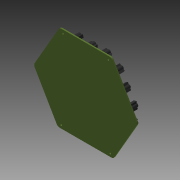
# Autodesk Inventor part: PCB
Saved by Autodesk Inventor 2015 (Build 190159000, 159)
## iProperties
Created: 2016-10-01
Part Number: PCB
Material: Generic
Document SubType Name: Modeling
Designer: James Yelland
Density: 1 g/cm^3
Appearance: Default
Author: James Yelland
Autodesk Inventor part; units mm, degrees
ref_plane "YZ Plane" through (0, 0, 0) normal (1, 0, 0) x (0, 1, 0)
ref_plane "XZ Plane" through (0, 0, 0) normal (0, 1, 0) x (-1, 0, 0)
ref_plane "XY Plane" through (0, 0, 0) normal (0, 0, 1) x (1, 0, 0)
sketch "Sketch1" plane through (0, 0, 0) normal (0, 1, 0) x (-1, 0, 0)
  line L0 (-78.5566, 2.5) -> (-41.4434, 66.782)
  line L1 (-37.1132, 69.282) -> (37.1132, 69.282)
  line L2 (41.4434, 66.782) -> (78.5566, 2.5)
  line L3 (0, -64.282) -> (-40, -64.282)
  line L4 (0, -64.282) -> (40, -64.282)
  line L5 (78.5566, -2.5) -> (44.3301, -61.782)
  line L6 (-44.3301, -61.782) -> (-78.5566, -2.5)
  arc A0 (78.5566, -2.5) -> (78.5566, 2.5) centre (74.2265, 0) ccw
  arc A1 (40, -64.282) -> (44.3301, -61.782) centre (40, -59.282) ccw
  arc A2 (-44.3301, -61.782) -> (-40, -64.282) centre (-40, -59.282) ccw
  arc A3 (-78.5566, 2.5) -> (-78.5566, -2.5) centre (-74.2265, 0) ccw
  arc A4 (-37.1132, 69.282) -> (-41.4434, 66.782) centre (-37.1132, 64.282) ccw
  arc A5 (41.4434, 66.782) -> (37.1132, 69.282) centre (37.1132, 64.282) ccw
  circle A6 centre (37.937, -59.3323) radius 1.6
  circle A7 centre (-37.937, -59.3323) radius 1.6
  circle A8 centre (-35.0503, 64.3323) radius 1.6
  circle A9 centre (35.0503, 64.3323) radius 1.6
  point P0 (80, 0)
  point P1 (-80, 0)
  point P2 (-42.8868, -64.282)
  point P3 (42.8868, -64.282)
  dimension "d21" = 5
  dimension "d35" = 3.2
  dimension "d38" = 3.2
  dimension "d45" = 3.2
  dimension "d46" = 3.2
  constraints: 14 end point, 12 point on circle, 12 tangent, 10 centre point, 9 point on line, 5 equal radius
  measures "d21" radius of A0
  measures "d35" diameter of A6
  measures "d38" diameter of A7
  measures "d45" diameter of A8
  measures "d46" diameter of A9
extrude "Extrusion1" add sketch "Sketch1" along normal blind 2
sketch "Sketch4" plane through (0, 2, 0) normal (0, 1, 0) x (1, 0, 0)
  line L0 (5, 57.282) -> (5, 53.282)
  arc A0 (2.5807, 57.282) -> (-2.5807, 57.282) centre (0, 56.332) ccw
  line L1 (-5, 57.282) -> (-2.5807, 57.282)
  line L2 (5, 53.282) -> (-5, 53.282)
  line L3 (-5, 53.282) -> (-5, 57.282)
  line L4 (2.5807, 57.282) -> (5, 57.282)
  line L5 (-24.333, 52.2353) -> (-25.7011, 55.9941)
  line L6 (-25.7011, 55.9941) -> (-23.4277, 56.8215)
  arc A1 (-18.5775, 58.5868) -> (-23.4277, 56.8215) centre (-20.6777, 56.8115) ccw
  line L7 (-14.9361, 55.6555) -> (-24.333, 52.2353)
  line L8 (-16.3041, 59.4143) -> (-14.9361, 55.6555)
  line L9 (-18.5775, 58.5868) -> (-16.3041, 59.4143)
  line L10 (-44.1513, 44.8388) -> (-46.7224, 47.903)
  line L11 (-46.7224, 47.903) -> (-44.8691, 49.4581)
  arc A2 (-40.9153, 52.7758) -> (-44.8691, 49.4581) centre (-42.2815, 50.3892) ccw
  line L12 (-36.4908, 51.2667) -> (-44.1513, 44.8388)
  line L13 (-39.062, 54.3309) -> (-36.4908, 51.2667)
  line L14 (-40.9153, 52.7758) -> (-39.062, 54.3309)
  line L15 (-52.9737, 24.8109) -> (-56.4378, 26.8109)
  line L16 (-56.4378, 26.8109) -> (-55.2282, 28.9061)
  arc A3 (-52.6475, 33.376) -> (-55.2282, 28.9061) centre (-53.1151, 30.666) ccw
  line L17 (-47.9737, 33.4711) -> (-52.9737, 24.8109)
  line L18 (-51.4378, 35.4711) -> (-47.9737, 33.4711)
  line L19 (-52.6475, 33.376) -> (-51.4378, 35.4711)
  line L20 (-62.6437, 5.9686) -> (-66.5829, 6.6632)
  line L21 (-66.5829, 6.6632) -> (-66.1628, 9.0458)
  arc A4 (-65.2665, 14.1288) -> (-66.1628, 9.0458) centre (-64.7791, 11.4223) ccw
  line L22 (-60.9072, 15.8167) -> (-62.6437, 5.9686)
  line L23 (-64.8464, 16.5113) -> (-60.9072, 15.8167)
  line L24 (-65.2665, 14.1288) -> (-64.8464, 16.5113)
  line L25 (-60.9072, -15.8167) -> (-64.8464, -16.5113)
  line L26 (-64.8464, -16.5113) -> (-65.2665, -14.1288)
  arc A5 (-66.1628, -9.0458) -> (-65.2665, -14.1288) centre (-64.7791, -11.4223) ccw
  line L27 (-62.6437, -5.9686) -> (-60.9072, -15.8167)
  line L28 (-66.5829, -6.6632) -> (-62.6437, -5.9686)
  line L29 (-66.1628, -9.0458) -> (-66.5829, -6.6632)
  line L30 (-47.9737, -33.4711) -> (-51.4378, -35.4711)
  line L31 (-51.4378, -35.4711) -> (-52.6475, -33.376)
  arc A6 (-55.2282, -28.9061) -> (-52.6475, -33.376) centre (-53.1151, -30.666) ccw
  line L32 (-52.9737, -24.8109) -> (-47.9737, -33.4711)
  line L33 (-56.4378, -26.8109) -> (-52.9737, -24.8109)
  line L34 (-55.2282, -28.9061) -> (-56.4378, -26.8109)
  line L35 (-36.4908, -51.2667) -> (-39.062, -54.3309)
  line L36 (-39.062, -54.3309) -> (-40.9153, -52.7758)
  arc A7 (-44.8691, -49.4581) -> (-40.9153, -52.7758) centre (-42.2815, -50.3892) ccw
  line L37 (-44.1513, -44.8388) -> (-36.4908, -51.2667)
  line L38 (-46.7224, -47.903) -> (-44.1513, -44.8388)
  line L39 (-44.8691, -49.4581) -> (-46.7224, -47.903)
  line L40 (-16.7559, -60.6555) -> (-18.124, -64.4143)
  line L41 (-18.124, -64.4143) -> (-20.3974, -63.5868)
  arc A8 (-25.2475, -61.8215) -> (-20.3974, -63.5868) centre (-22.4975, -61.8115) ccw
  line L42 (-26.1528, -57.2353) -> (-16.7559, -60.6555)
  line L43 (-27.5209, -60.9941) -> (-26.1528, -57.2353)
  line L44 (-25.2475, -61.8215) -> (-27.5209, -60.9941)
  line L45 (5, -58.282) -> (5, -62.282)
  line L46 (5, -62.282) -> (2.5807, -62.282)
  arc A9 (-2.5807, -62.282) -> (2.5807, -62.282) centre (0, -61.332) ccw
  line L47 (-5, -58.282) -> (5, -58.282)
  line L48 (-5, -62.282) -> (-5, -58.282)
  line L49 (-2.5807, -62.282) -> (-5, -62.282)
  line L50 (26.1528, -57.2353) -> (27.5209, -60.9941)
  line L51 (27.5209, -60.9941) -> (25.2475, -61.8215)
  arc A10 (20.3974, -63.5868) -> (25.2475, -61.8215) centre (22.4975, -61.8115) ccw
  line L52 (16.7559, -60.6555) -> (26.1528, -57.2353)
  line L53 (18.124, -64.4143) -> (16.7559, -60.6555)
  line L54 (20.3974, -63.5868) -> (18.124, -64.4143)
  line L55 (44.1513, -44.8388) -> (46.7224, -47.903)
  line L56 (46.7224, -47.903) -> (44.8691, -49.4581)
  arc A11 (40.9153, -52.7758) -> (44.8691, -49.4581) centre (42.2815, -50.3892) ccw
  line L57 (36.4908, -51.2667) -> (44.1513, -44.8388)
  line L58 (39.062, -54.3309) -> (36.4908, -51.2667)
  line L59 (40.9153, -52.7758) -> (39.062, -54.3309)
  line L60 (52.9737, -24.8109) -> (56.4378, -26.8109)
  line L61 (56.4378, -26.8109) -> (55.2282, -28.9061)
  arc A12 (52.6475, -33.376) -> (55.2282, -28.9061) centre (53.1151, -30.666) ccw
  line L62 (47.9737, -33.4711) -> (52.9737, -24.8109)
  line L63 (51.4378, -35.4711) -> (47.9737, -33.4711)
  line L64 (52.6475, -33.376) -> (51.4378, -35.4711)
  line L65 (62.6437, -5.9686) -> (66.5829, -6.6632)
  line L66 (66.5829, -6.6632) -> (66.1628, -9.0458)
  arc A13 (65.2665, -14.1288) -> (66.1628, -9.0458) centre (64.7791, -11.4223) ccw
  line L67 (60.9072, -15.8167) -> (62.6437, -5.9686)
  line L68 (64.8464, -16.5113) -> (60.9072, -15.8167)
  line L69 (65.2665, -14.1288) -> (64.8464, -16.5113)
  line L70 (60.9072, 15.8167) -> (64.8464, 16.5113)
  line L71 (64.8464, 16.5113) -> (65.2665, 14.1288)
  arc A14 (66.1628, 9.0458) -> (65.2665, 14.1288) centre (64.7791, 11.4223) ccw
  line L72 (62.6437, 5.9686) -> (60.9072, 15.8167)
  line L73 (66.5829, 6.6632) -> (62.6437, 5.9686)
  line L74 (66.1628, 9.0458) -> (66.5829, 6.6632)
  line L75 (47.9737, 33.4711) -> (51.4378, 35.4711)
  line L76 (51.4378, 35.4711) -> (52.6475, 33.376)
  arc A15 (55.2282, 28.9061) -> (52.6475, 33.376) centre (53.1151, 30.666) ccw
  line L77 (52.9737, 24.8109) -> (47.9737, 33.4711)
  line L78 (56.4378, 26.8109) -> (52.9737, 24.8109)
  line L79 (55.2282, 28.9061) -> (56.4378, 26.8109)
  line L80 (36.4908, 51.2667) -> (39.062, 54.3309)
  line L81 (39.062, 54.3309) -> (40.9153, 52.7758)
  arc A16 (44.8691, 49.4581) -> (40.9153, 52.7758) centre (42.2815, 50.3892) ccw
  line L82 (44.1513, 44.8388) -> (36.4908, 51.2667)
  line L83 (46.7224, 47.903) -> (44.1513, 44.8388)
  line L84 (44.8691, 49.4581) -> (46.7224, 47.903)
  line L85 (14.9361, 55.6555) -> (16.3041, 59.4143)
  line L86 (16.3041, 59.4143) -> (18.5775, 58.5868)
  arc A17 (23.4277, 56.8215) -> (18.5775, 58.5868) centre (20.6777, 56.8115) ccw
  line L87 (24.333, 52.2353) -> (14.9361, 55.6555)
  line L88 (25.7011, 55.9941) -> (24.333, 52.2353)
  line L89 (23.4277, 56.8215) -> (25.7011, 55.9941)
  line L90 (40, 64.282) -> (-40, 64.282) projected
  arc A18 (-40, 64.282) -> (-44.3301, 61.782) centre (-40, 59.282) ccw projected
  line L91 (-44.3301, 61.782) -> (-78.5566, 2.5) projected
  arc A19 (-78.5566, 2.5) -> (-78.5566, -2.5) centre (-74.2265, 0) ccw projected
  line L92 (-78.5566, -2.5) -> (-41.4434, -66.782) projected
  arc A20 (-41.4434, -66.782) -> (-37.1132, -69.282) centre (-37.1132, -64.282) ccw projected
  line L93 (-37.1132, -69.282) -> (37.1132, -69.282) projected
  arc A21 (37.1132, -69.282) -> (41.4434, -66.782) centre (37.1132, -64.282) ccw projected
  line L94 (41.4434, -66.782) -> (78.5566, -2.5) projected
  arc A22 (78.5566, -2.5) -> (78.5566, 2.5) centre (74.2265, 0) ccw projected
  line L95 (78.5566, 2.5) -> (44.3301, 61.782) projected
  arc A23 (44.3301, 61.782) -> (40, 64.282) centre (40, 59.282) ccw projected
  line L96 (40, 64.282) -> (-40, 64.282) projected
  line L97 (44.3301, 61.782) -> (78.5566, 2.5) projected
  line L98 (41.4434, -66.782) -> (78.5566, -2.5) projected
  line L99 (37.1132, -69.282) -> (-37.1132, -69.282) projected
  line L100 (-41.4434, -66.782) -> (-78.5566, -2.5) projected
  line L101 (78.5566, 2.5) -> (44.3301, 61.782) projected
  line L102 (-78.5566, 2.5) -> (-44.3301, 61.782) projected
  dimension "d24" = 360
  constraints: 180 end point, 36 point on circle, 18 centre point
extrude "Extrusion4" add sketch "Sketch4" along normal blind 12 contours L0 L2 L3 L1 A0 L4 | L5 L6 A1 L9 L8 L7 | L10 L11 A2 L14 L13 L12 | L15 L16 A3 L19 L18 L17 | L20 L21 A4 L24 L23 L22 | L25 L26 A5 L29 L28 L27 | L30 L31 A6 L34 L33 L32 | L35 L36 A7 L39 L38 L37 | L40 L41 A8 L44 L43 L42 | L45 L46 A9 L49 L48 L47 | L50 L51 A10 L54 L53 L52 | L55 L56 A11 L59 L58 L57 | L60 L61 A12 L64 L63 L62 | L65 L66 A13 L69 L68 L67 | L70 L71 A14 L74 L73 L72 | L75 L76 A15 L79 L78 L77 | L80 L81 A16 L84 L83 L82 | L85 L86 A17 L89 L88 L87
body "Solid1"
